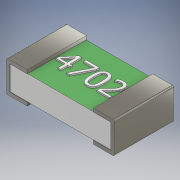
# Autodesk Inventor part: 21-1001
Saved by Autodesk Inventor 2018 (Build 220112000, 112)
## iProperties
Created: 2019-09-21
Part Number: 21-1001
Material: Copper
Document SubType Name: Modeling
Designer: Bradley
Density: 8.94 g/cm^3
Appearance: Smooth - White
Author: Bradley
Autodesk Inventor part; units mm, degrees
ref_plane "YZ Plane" through (0, 0, 0) normal (1, 0, 0) x (0, 1, 0)
ref_plane "XZ Plane" through (0, 0, 0) normal (0, 1, 0) x (-1, 0, 0)
ref_plane "XY Plane" through (0, 0, 0) normal (0, 0, 1) x (1, 0, 0)
sketch "Sketch1" plane through (0, 0, 0) normal (0, 1, 0) x (-1, 0, 0)
  line L0 (0.725, 0.175) -> (-0.725, 0.175)
  line L1 (-0.725, 0.175) -> (-0.725, -0.175)
  line L2 (-0.725, -0.175) -> (0.725, -0.175)
  line L3 (0.725, -0.175) -> (0.725, 0.175)
  line L4 (0.475, 0.175) -> (0.475, 0.225)
  line L5 (0.475, 0.225) -> (0.775, 0.225)
  line L6 (0.775, 0.225) -> (0.775, -0.225)
  line L7 (0.775, -0.225) -> (0.475, -0.225)
  line L8 (0.475, -0.225) -> (0.475, -0.175)
  line L9 (-0.475, 0.175) -> (-0.475, 0.225)
  line L10 (-0.475, 0.225) -> (-0.775, 0.225)
  line L11 (-0.775, 0.225) -> (-0.775, -0.225)
  line L12 (-0.775, -0.225) -> (-0.475, -0.225)
  line L13 (-0.475, -0.175) -> (-0.475, -0.225)
  line L14 (0.475, 0.175) -> (-0.475, 0.175)
  point P0 (0, 0)
  point P1 (0, 0.175)
  point P2 (0.725, 0)
  dimension "d0" = 1.55
  dimension "d1" = 0.05
  dimension "d2" = 0.05
  dimension "d3" = 0.45
  dimension "d4" = 0.3
  constraints: 30 end point, 12 point on line, 7 perpendicular, 3 collinear, 3 midpoint, 2 parallel, 1 horizontal, 1 horizontal alignment, 1 vertical, 1 vertical alignment
  measures "d0" distance between parallel lines of L11 L6
  measures "d1" distance of L7.end L8.end
  measures "d2" distance between parallel lines of L6 L3
  measures "d3" distance of L5.end L6.end
  measures "d4" distance of L6.end L7.end
extrude "Extrusion1" add sketch "Sketch1" along normal mid plane 0.85 contours L0 L4 L5 L6 L7 L8 L2 L3 | L0 L1 L2 L13 L12 L11 L10 L9
extrude "Extrusion2" add sketch "Sketch1" along normal mid plane 0.84 contours L3 L2 L1 L0
sketch "Sketch2" plane through (-0.475, -0.42, 0.175) normal (0, 0, 1) x (1, 0, 0)
  line L0 (0, 0) -> (0, 0.84) projected
  line L1 (0.95, 0) -> (0, 0) projected
  line L2 (0.95, 0) -> (0.95, 0.84) projected
  line L3 (0, 0.84) -> (0.95, 0.84) projected
  line L4 (0, 0.42) -> (0.95, 0.42) construction
  line L5 (0.2397, 0.3731) -> (0.2039, 0.3731)
  line L6 (0.2039, 0.3731) -> (0.2039, 0.27)
  line L7 (0.2039, 0.27) -> (0.1653, 0.27)
  line L8 (0.1653, 0.27) -> (0.1653, 0.3731)
  line L9 (0.1653, 0.3731) -> (0.0328, 0.3731)
  line L10 (0.0328, 0.3731) -> (0.0328, 0.4154)
  line L11 (0.0328, 0.4154) -> (0.167, 0.57)
  line L12 (0.167, 0.57) -> (0.2039, 0.57)
  line L13 (0.2039, 0.57) -> (0.2039, 0.4054)
  line L14 (0.2039, 0.4054) -> (0.2397, 0.4054)
  line L15 (0.2397, 0.4054) -> (0.2397, 0.3731)
  line L16 (0.1653, 0.4054) -> (0.1653, 0.5226)
  line L17 (0.1653, 0.5226) -> (0.0644, 0.4054)
  line L18 (0.0644, 0.4054) -> (0.1653, 0.4054)
  line L19 (0.4602, 0.525) -> (0.3303, 0.27)
  line L20 (0.3303, 0.27) -> (0.2876, 0.27)
  line L21 (0.2876, 0.27) -> (0.4247, 0.5347)
  line L22 (0.4247, 0.5347) -> (0.2698, 0.5347)
  line L23 (0.2698, 0.5347) -> (0.2698, 0.57)
  line L24 (0.2698, 0.57) -> (0.4602, 0.57)
  line L25 (0.4602, 0.57) -> (0.4602, 0.525)
  spline S0 degree 2 poles (0.6836, 0.42) (0.6836, 0.3393) (0.6367, 0.2637) (0.5878, 0.2637) knots 0 0 0 1 2 2 2
  spline S1 degree 2 poles (0.5878, 0.2637) (0.5382, 0.2637) (0.4918, 0.3407) (0.4918, 0.4198) knots 0 0 0 1 2 2 2
  spline S2 degree 2 poles (0.4918, 0.4198) (0.4918, 0.501) (0.5387, 0.5761) (0.5878, 0.5761) knots 0 0 0 1 2 2 2
  spline S3 degree 2 poles (0.5878, 0.5761) (0.6372, 0.5761) (0.6836, 0.4983) (0.6836, 0.42) knots 0 0 0 1 2 2 2
  spline S4 degree 2 poles (0.6321, 0.3286) (0.6379, 0.3434) (0.6427, 0.3891) (0.6427, 0.42) knots 0 0 0 1 2 2 2
  spline S5 degree 2 poles (0.6427, 0.42) (0.6427, 0.4509) (0.6379, 0.4963) (0.6318, 0.5117) knots 0 0 0 1 2 2 2
  spline S6 degree 2 poles (0.6318, 0.5117) (0.6257, 0.527) (0.6046, 0.5428) (0.5878, 0.5428) knots 0 0 0 1 2 2 2
  spline S7 degree 2 poles (0.5878, 0.5428) (0.571, 0.5428) (0.5494, 0.527) (0.5431, 0.5112) knots 0 0 0 1 2 2 2
  spline S8 degree 2 poles (0.5431, 0.5112) (0.537, 0.4959) (0.5326, 0.4492) (0.5326, 0.4198) knots 0 0 0 1 2 2 2
  spline S9 degree 2 poles (0.5326, 0.4198) (0.5326, 0.3882) (0.5365, 0.3459) (0.5428, 0.3293) knots 0 0 0 1 2 2 2
  spline S10 degree 2 poles (0.5428, 0.3293) (0.5487, 0.3138) (0.5703, 0.297) (0.5878, 0.297) knots 0 0 0 1 2 2 2
  spline S11 degree 2 poles (0.5878, 0.297) (0.6043, 0.297) (0.626, 0.3128) (0.6321, 0.3286) knots 0 0 0 1 2 2 2
  line L26 (0.907, 0.27) -> (0.722, 0.27)
  line L27 (0.722, 0.27) -> (0.722, 0.3125)
  spline S12 degree 2 poles (0.722, 0.3125) (0.7419, 0.3313) (0.7774, 0.366) (0.7944, 0.3847) knots 0 0 0 1 2 2 2
  spline S13 degree 2 poles (0.7944, 0.3847) (0.8287, 0.4224) (0.8538, 0.4676) (0.8538, 0.4917) knots 0 0 0 1 2 2 2
  spline S14 degree 2 poles (0.8538, 0.4917) (0.8538, 0.5044) (0.846, 0.5233) (0.8389, 0.5294) knots 0 0 0 1 2 2 2
  spline S15 degree 2 poles (0.8389, 0.5294) (0.8319, 0.5355) (0.8134, 0.5416) (0.8022, 0.5416) knots 0 0 0 1 2 2 2
  spline S16 degree 2 poles (0.8022, 0.5416) (0.7915, 0.5416) (0.7697, 0.5362) (0.7597, 0.5321) knots 0 0 0 1 2 2 2
  spline S17 degree 2 poles (0.7597, 0.5321) (0.7512, 0.5287) (0.7354, 0.5189) (0.7305, 0.5155) knots 0 0 0 1 2 2 2
  line L28 (0.7305, 0.5155) -> (0.7283, 0.5155)
  line L29 (0.7283, 0.5155) -> (0.7283, 0.5583)
  spline S18 degree 2 poles (0.7283, 0.5583) (0.7407, 0.5644) (0.7852, 0.5763) (0.8051, 0.5763) knots 0 0 0 1 2 2 2
  spline S19 degree 2 poles (0.8051, 0.5763) (0.8472, 0.5763) (0.8946, 0.5318) (0.8946, 0.4939) knots 0 0 0 1 2 2 2
  spline S20 degree 2 poles (0.8946, 0.4939) (0.8946, 0.4762) (0.8863, 0.4465) (0.8791, 0.4339) knots 0 0 0 1 2 2 2
  spline S21 degree 2 poles (0.8791, 0.4339) (0.8718, 0.4207) (0.8506, 0.395) (0.8389, 0.3826) knots 0 0 0 1 2 2 2
  spline S22 degree 2 poles (0.8389, 0.3826) (0.82, 0.3619) (0.7735, 0.3176) (0.7597, 0.3048) knots 0 0 0 1 2 2 2
  line L30 (0.7597, 0.3048) -> (0.907, 0.3048)
  line L31 (0.907, 0.3048) -> (0.907, 0.27)
  point P0 (0.475, 0.42)
  constraints: 2 end point, 2 midpoint, 1 horizontal
extrude "Extrusion3" add sketch "Sketch2" along normal blind 0.02 contours L5 L6 L7 L8 L9 L10 L11 L12 L13 L14 L15 | L19 L20 L21 L22 L23 L24 L25 | S0 S1 S2 S3 | L26 L27 S12 S13 S14 S15 S16 S17 L28 L29 S18 S19 S20 S21 S22 L30 L31
fillet "Fillet1" radius 0.02 4 edges at (-0.775, 0, 0.225) (-0.775, 0, -0.225) (0.775, 0, 0.225) (0.775, 0, -0.225)
equation "\"d2\" = d1"
body "Solid1"
